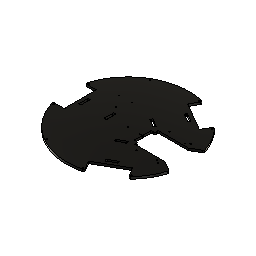
LowerPlate v13 (Autodesk Fusion 360 design; units mm, degrees)
Autodesk Fusion 360 part; units mm, degrees
(part 1 of 2)
sketch "Sketch1" plane through (0, 0, 0) normal (0, 0, 1) x (1, 0, 0)
  line L0 (0, 0) -> (-132.5, 0) construction
  line L1 (0, 0) -> (132.5, 0) construction
  line L2 (0, 0) -> (66.25, 114.7484) construction
  line L3 (0, 0) -> (66.25, -114.7484) construction
  line L4 (-127.7938, -35) -> (-103.7938, -35) construction
  line L5 (-103.7938, -35) -> (-103.7938, 35) construction
  line L6 (-103.7938, 35) -> (-127.7938, 35) construction
  line L7 (-127.7938, 35) -> (-127.7938, -35) construction
  line L8 (-103.7938, 35) -> (-104.8544, 33.9393) construction
  line L9 (-103.7938, -35) -> (-104.8544, -33.9393) construction
  arc A0 (-124.4739, -35) -> (-126.8676, -38.2212) centre (-124.4739, -37.5) ccw
  arc A1 (-126.8676, -38.2212) -> (-124.4739, -35) centre (-124.4739, -37.5) ccw construction
  arc A2 (-103.7938, -35) -> (-103.7938, -32.8787) centre (-104.8544, -33.9393) ccw
  arc A3 (-103.7938, -32.8787) -> (-105.9151, -35) centre (-104.8544, -33.9393) ccw construction
  arc A4 (-105.9151, -35) -> (-103.7938, -35) centre (-104.8544, -33.9393) ccw
  arc A5 (-103.7938, 32.8787) -> (-105.9151, 35) centre (-104.8544, 33.9393) ccw
  arc A6 (-105.9151, 35) -> (-103.7938, 32.8787) centre (-104.8544, 33.9393) ccw construction
  arc A7 (-126.8676, 38.2212) -> (-124.4739, 35) centre (-124.4739, 37.5) ccw
  arc A8 (-124.4739, 35) -> (-126.8676, 38.2212) centre (-124.4739, 37.5) ccw construction
  line L10 (-124.4739, 35) -> (-105.9151, 35)
  line L11 (-103.7938, 32.8787) -> (-103.7938, -32.8787)
  line L12 (-105.9151, -35) -> (-124.4739, -35)
  line L13 (33.586, 128.1727) -> (94.2078, 93.1727) construction
  line L14 (33.586, 128.1727) -> (21.586, 107.388) construction
  line L15 (21.586, 107.388) -> (82.2078, 72.388) construction
  line L16 (82.2078, 72.388) -> (94.2078, 93.1727) construction
  arc A9 (31.9261, 125.2976) -> (30.3332, 128.9812) centre (29.761, 126.5476) ccw
  arc A10 (30.3332, 128.9812) -> (31.9261, 125.2976) centre (29.761, 126.5476) ccw construction
  arc A11 (96.5343, 90.76) -> (92.5478, 90.2976) centre (94.7129, 89.0476) ccw
  arc A12 (92.5478, 90.2976) -> (96.5343, 90.76) centre (94.7129, 89.0476) ccw construction
  line L17 (21.586, 107.388) -> (23.0349, 107.7763) construction
  arc A13 (22.6467, 109.2252) -> (23.4231, 106.3274) centre (23.0349, 107.7763) ccw
  arc A14 (23.4231, 106.3274) -> (22.6467, 109.2252) centre (23.0349, 107.7763) ccw construction
  line L18 (82.2078, 72.388) -> (81.8196, 73.8369) construction
  arc A15 (80.3707, 73.4487) -> (83.2684, 74.2252) centre (81.8196, 73.8369) ccw
  arc A16 (83.2684, 74.2252) -> (80.3707, 73.4487) centre (81.8196, 73.8369) ccw construction
  line L19 (83.2684, 74.2252) -> (92.5478, 90.2976)
  line L20 (80.3707, 73.4487) -> (23.4231, 106.3274)
  line L21 (22.6467, 109.2252) -> (31.9261, 125.2976)
  line L22 (33.586, -128.1727) -> (94.2078, -93.1727) construction
  line L23 (33.586, -128.1727) -> (21.586, -107.388) construction
  line L24 (21.586, -107.388) -> (82.2078, -72.388) construction
  line L25 (82.2078, -72.388) -> (94.2078, -93.1727) construction
  line L26 (82.2078, -72.388) -> (81.8196, -73.8369) construction
  line L27 (21.586, -107.388) -> (23.0349, -107.7763) construction
  arc A17 (23.4231, -106.3274) -> (22.6467, -109.2252) centre (23.0349, -107.7763) ccw
  arc A18 (22.6467, -109.2252) -> (23.4231, -106.3274) centre (23.0349, -107.7763) ccw construction
  arc A19 (83.2684, -74.2252) -> (80.3707, -73.4487) centre (81.8196, -73.8369) ccw
  arc A20 (80.3707, -73.4487) -> (83.2684, -74.2252) centre (81.8196, -73.8369) ccw construction
  arc A21 (92.5478, -90.2976) -> (96.5343, -90.76) centre (94.7129, -89.0476) ccw
  arc A22 (96.5343, -90.76) -> (92.5478, -90.2976) centre (94.7129, -89.0476) ccw construction
  arc A23 (30.3333, -128.9812) -> (31.9261, -125.2976) centre (29.761, -126.5476) ccw
  arc A24 (31.9261, -125.2976) -> (30.3333, -128.9812) centre (29.761, -126.5476) ccw construction
  line L28 (92.5478, -90.2976) -> (83.2684, -74.2252)
  line L29 (80.3707, -73.4487) -> (23.4231, -106.3274)
  line L30 (22.6467, -109.2252) -> (31.9261, -125.2976)
  arc A25 (30.3332, 128.9812) -> (-126.8676, 38.2212) centre (0, 0) ccw
  arc A26 (-126.8676, 38.2212) -> (-126.8676, -38.2212) centre (0, 0) ccw construction
  arc A27 (30.3333, -128.9812) -> (30.3332, 128.9812) centre (0, 0) ccw construction
  arc A28 (-126.8676, -38.2212) -> (30.3333, -128.9812) centre (0, 0) ccw
  line L31 (-103.7938, 18.4) -> (-19.3938, 18.4) construction
  line L32 (-19.3938, 18.4) -> (-19.3938, -18.4) construction
  line L33 (-19.3938, -18.4) -> (-103.7938, -18.4) construction
  line L34 (-96.7938, 10) -> (-91.9938, 10) construction
  line L35 (-91.9938, 10) -> (-91.9938, -10) construction
  line L36 (-91.9938, -10) -> (-96.7938, -10) construction
  line L37 (-96.7938, -10) -> (-96.7938, 10) construction
  line L38 (-96.7938, 10) -> (-91.9938, -10) construction
  line L39 (-41.9938, 10) -> (-37.1938, 10) construction
  line L40 (-37.1938, 10) -> (-37.1938, -10) construction
  line L41 (-37.1938, -10) -> (-41.9938, -10) construction
  line L42 (-41.9938, -10) -> (-41.9938, 10) construction
  line L43 (-41.9938, 10) -> (-37.1938, -10) construction
  line L44 (-96.7938, 10) -> (-95.7331, 8.9393) construction
  line L45 (-91.9938, 10) -> (-93.0544, 8.9393) construction
  line L46 (-96.7938, -10) -> (-95.7331, -8.9393) construction
  line L47 (-91.9938, -10) -> (-93.0544, -8.9393) construction
  arc A29 (-94.1151, 10) -> (-91.9938, 7.8787) centre (-93.0544, 8.9393) ccw construction
  arc A30 (-91.9938, 7.8787) -> (-91.9938, 10) centre (-93.0544, 8.9393) ccw
  arc A31 (-91.9938, 10) -> (-94.1151, 10) centre (-93.0544, 8.9393) ccw
  arc A32 (-96.7938, 7.8787) -> (-94.6725, 10) centre (-95.7331, 8.9393) ccw construction
  arc A33 (-94.6725, 10) -> (-96.7938, 10) centre (-95.7331, 8.9393) ccw
  arc A34 (-96.7938, 10) -> (-96.7938, 7.8787) centre (-95.7331, 8.9393) ccw
  arc A35 (-94.6725, -10) -> (-96.7938, -7.8787) centre (-95.7331, -8.9393) ccw construction
  arc A36 (-96.7938, -7.8787) -> (-96.7938, -10) centre (-95.7331, -8.9393) ccw
  arc A37 (-96.7938, -10) -> (-94.6725, -10) centre (-95.7331, -8.9393) ccw
  arc A38 (-91.9938, -7.8787) -> (-94.1151, -10) centre (-93.0544, -8.9393) ccw construction
  arc A39 (-94.1151, -10) -> (-91.9938, -10) centre (-93.0544, -8.9393) ccw
  arc A40 (-91.9938, -10) -> (-91.9938, -7.8787) centre (-93.0544, -8.9393) ccw
  line L48 (-94.6725, 10) -> (-94.1151, 10)
  line L49 (-96.7938, 7.8787) -> (-96.7938, -7.8787)
  line L50 (-91.9938, -7.8787) -> (-91.9938, 7.8787)
  line L51 (-94.6725, -10) -> (-94.1151, -10)
  line L52 (-41.9938, 10) -> (-40.9331, 8.9393) construction
  line L53 (-37.1938, 10) -> (-38.2544, 8.9393) construction
  line L54 (-41.9938, -10) -> (-40.9331, -8.9393) construction
  line L55 (-37.1938, -10) -> (-38.2544, -8.9393) construction
  arc A41 (-37.1938, -7.8787) -> (-39.3151, -10) centre (-38.2544, -8.9393) ccw construction
  arc A42 (-39.3151, -10) -> (-37.1938, -10) centre (-38.2544, -8.9393) ccw
  arc A43 (-37.1938, -10) -> (-37.1938, -7.8787) centre (-38.2544, -8.9393) ccw
  arc A44 (-39.8725, -10) -> (-41.9938, -7.8787) centre (-40.9331, -8.9393) ccw construction
  arc A45 (-41.9938, -10) -> (-39.8725, -10) centre (-40.9331, -8.9393) ccw
  arc A46 (-41.9938, -7.8787) -> (-41.9938, -10) centre (-40.9331, -8.9393) ccw
  arc A47 (-41.9938, 7.8787) -> (-39.8725, 10) centre (-40.9331, 8.9393) ccw construction
  arc A48 (-41.9938, 10) -> (-41.9938, 7.8787) centre (-40.9331, 8.9393) ccw
  arc A49 (-39.8725, 10) -> (-41.9938, 10) centre (-40.9331, 8.9393) ccw
  arc A50 (-39.3151, 10) -> (-37.1938, 7.8787) centre (-38.2544, 8.9393) ccw construction
  arc A51 (-37.1938, 10) -> (-39.3151, 10) centre (-38.2544, 8.9393) ccw
  arc A52 (-37.1938, 7.8787) -> (-37.1938, 10) centre (-38.2544, 8.9393) ccw
  line L56 (-39.8725, -10) -> (-39.3151, -10)
  line L57 (-37.1938, -7.8787) -> (-37.1938, 7.8787)
  line L58 (-41.9938, 7.8787) -> (-41.9938, -7.8787)
  line L59 (-39.8725, 10) -> (-39.3151, 10)
  line L60 (35.962, 99.088) -> (-6.238, 25.9955) construction
  line L61 (-6.238, 25.9955) -> (25.6318, 7.5955) construction
  line L62 (25.6318, 7.5955) -> (67.8318, 80.688) construction
  line L63 (39.7366, 88.8259) -> (57.0571, 78.8259) construction
  line L64 (57.0571, 78.8259) -> (54.6571, 74.6689) construction
  line L65 (54.6571, 74.6689) -> (37.3366, 84.6689) construction
  line L66 (37.3366, 84.6689) -> (39.7366, 88.8259) construction
  line L67 (39.7366, 88.8259) -> (54.6571, 74.6689) construction
  line L68 (12.3366, 41.3677) -> (29.6571, 31.3677) construction
  line L69 (29.6571, 31.3677) -> (27.2571, 27.2108) construction
  line L70 (27.2571, 27.2108) -> (9.9366, 37.2108) construction
  line L71 (9.9366, 37.2108) -> (12.3366, 41.3677) construction
  line L72 (12.3366, 41.3677) -> (27.2571, 27.2108) construction
  line L73 (37.3366, 84.6689) -> (38.7855, 85.0572) construction
  line L74 (39.7366, 88.8259) -> (40.1249, 87.377) construction
  line L75 (54.6571, 74.6689) -> (54.2689, 76.1178) construction
  line L76 (57.0571, 78.8259) -> (55.6083, 78.4376) construction
  arc A53 (55.22, 79.8865) -> (55.9965, 76.9888) centre (55.6083, 78.4376) ccw construction
  arc A54 (55.9965, 76.9888) -> (57.0571, 78.8259) centre (55.6083, 78.4376) ccw
  arc A55 (57.0571, 78.8259) -> (55.22, 79.8865) centre (55.6083, 78.4376) ccw
  arc A56 (55.7178, 76.5061) -> (52.82, 75.7296) centre (54.2689, 76.1178) ccw construction
  arc A57 (54.6571, 74.6689) -> (55.7178, 76.5061) centre (54.2689, 76.1178) ccw
  arc A58 (52.82, 75.7296) -> (54.6571, 74.6689) centre (54.2689, 76.1178) ccw
  arc A59 (39.1738, 83.6083) -> (38.3973, 86.5061) centre (38.7855, 85.0572) ccw construction
  arc A60 (37.3366, 84.6689) -> (39.1738, 83.6083) centre (38.7855, 85.0572) ccw
  arc A61 (38.3973, 86.5061) -> (37.3366, 84.6689) centre (38.7855, 85.0572) ccw
  arc A62 (38.676, 86.9888) -> (41.5738, 87.7652) centre (40.1249, 87.377) ccw construction
  arc A63 (41.5738, 87.7652) -> (39.7366, 88.8259) centre (40.1249, 87.377) ccw
  arc A64 (39.7366, 88.8259) -> (38.676, 86.9888) centre (40.1249, 87.377) ccw
  line L77 (38.3973, 86.5061) -> (38.676, 86.9888)
  line L78 (41.5738, 87.7652) -> (55.22, 79.8865)
  line L79 (55.9965, 76.9888) -> (55.7178, 76.5061)
  line L80 (52.82, 75.7296) -> (39.1738, 83.6083)
  line L81 (9.9366, 37.2108) -> (11.3855, 37.599) construction
  line L82 (12.3366, 41.3677) -> (12.7249, 39.9188) construction
  line L83 (27.2571, 27.2108) -> (26.8689, 28.6596) construction
  line L84 (29.6571, 31.3677) -> (28.2083, 30.9795) construction
  arc A65 (11.276, 39.5306) -> (14.1738, 40.307) centre (12.7249, 39.9188) ccw construction
  arc A66 (14.1738, 40.307) -> (12.3366, 41.3677) centre (12.7249, 39.9188) ccw
  arc A67 (12.3366, 41.3677) -> (11.276, 39.5306) centre (12.7249, 39.9188) ccw
  arc A68 (11.7738, 36.1501) -> (10.9973, 39.0479) centre (11.3855, 37.599) ccw construction
  arc A69 (10.9973, 39.0479) -> (9.9366, 37.2108) centre (11.3855, 37.599) ccw
  arc A70 (9.9366, 37.2108) -> (11.7738, 36.1501) centre (11.3855, 37.599) ccw
  arc A71 (28.3178, 29.0479) -> (25.42, 28.2714) centre (26.8689, 28.6596) ccw construction
  arc A72 (25.42, 28.2714) -> (27.2571, 27.2108) centre (26.8689, 28.6596) ccw
  arc A73 (27.2571, 27.2108) -> (28.3178, 29.0479) centre (26.8689, 28.6596) ccw
  arc A74 (27.82, 32.4283) -> (28.5965, 29.5306) centre (28.2083, 30.9795) ccw construction
  arc A75 (28.5965, 29.5306) -> (29.6571, 31.3677) centre (28.2083, 30.9795) ccw
  arc A76 (29.6571, 31.3677) -> (27.82, 32.4283) centre (28.2083, 30.9795) ccw
  line L85 (10.9973, 39.0479) -> (11.276, 39.5306)
  line L86 (11.7738, 36.1501) -> (25.42, 28.2714)
  line L87 (28.3178, 29.0479) -> (28.5965, 29.5306)
  line L88 (27.82, 32.4283) -> (14.1738, 40.307)
  line L89 (35.962, -99.088) -> (-6.238, -25.9955) construction
  line L90 (-6.238, -25.9955) -> (25.6318, -7.5955) construction
  line L91 (25.6318, -7.5955) -> (67.8318, -80.688) construction
  line L92 (39.7366, -88.8259) -> (57.0571, -78.8259) construction
  line L93 (57.0571, -78.8259) -> (54.6571, -74.6689) construction
  line L94 (54.6571, -74.6689) -> (37.3366, -84.6689) construction
  line L95 (37.3366, -84.6689) -> (39.7366, -88.8259) construction
  line L96 (37.3366, -84.6689) -> (57.0571, -78.8259) construction
  line L97 (12.3366, -41.3677) -> (29.6571, -31.3677) construction
  line L98 (29.6571, -31.3677) -> (27.2571, -27.2108) construction
  line L99 (27.2571, -27.2108) -> (9.9366, -37.2108) construction
  line L100 (9.9366, -37.2108) -> (12.3366, -41.3677) construction
  line L101 (9.9366, -37.2108) -> (29.6571, -31.3677) construction
  line L102 (9.9366, -37.2108) -> (11.3855, -37.599) construction
  line L103 (12.3366, -41.3677) -> (12.7249, -39.9188) construction
  line L104 (27.2571, -27.2108) -> (26.8689, -28.6596) construction
  line L105 (29.6571, -31.3677) -> (28.2083, -30.9795) construction
  arc A77 (25.42, -28.2714) -> (28.3178, -29.0479) centre (26.8689, -28.6596) ccw construction
  arc A78 (28.3178, -29.0479) -> (27.2571, -27.2108) centre (26.8689, -28.6596) ccw
  arc A79 (27.2571, -27.2108) -> (25.42, -28.2714) centre (26.8689, -28.6596) ccw
  arc A80 (28.5965, -29.5306) -> (27.82, -32.4283) centre (28.2083, -30.9795) ccw construction
  arc A81 (29.6571, -31.3677) -> (28.5965, -29.5306) centre (28.2083, -30.9795) ccw
  arc A82 (27.82, -32.4283) -> (29.6571, -31.3677) centre (28.2083, -30.9795) ccw
  arc A83 (14.1738, -40.307) -> (11.276, -39.5306) centre (12.7249, -39.9188) ccw construction
  arc A84 (12.3366, -41.3677) -> (14.1738, -40.307) centre (12.7249, -39.9188) ccw
  arc A85 (11.276, -39.5306) -> (12.3366, -41.3677) centre (12.7249, -39.9188) ccw
  arc A86 (10.9973, -39.0479) -> (11.7738, -36.1501) centre (11.3855, -37.599) ccw construction
  arc A87 (9.9366, -37.2108) -> (10.9973, -39.0479) centre (11.3855, -37.599) ccw
  arc A88 (11.7738, -36.1501) -> (9.9366, -37.2108) centre (11.3855, -37.599) ccw
  line L106 (28.5965, -29.5306) -> (28.3178, -29.0479)
  line L107 (25.42, -28.2714) -> (11.7738, -36.1501)
  line L108 (27.82, -32.4283) -> (14.1738, -40.307)
  line L109 (11.276, -39.5306) -> (10.9973, -39.0479)
  line L110 (37.3366, -84.6689) -> (38.7855, -85.0572) construction
  line L111 (39.7366, -88.8259) -> (40.1249, -87.377) construction
  line L112 (54.6571, -74.6689) -> (54.2689, -76.1178) construction
  line L113 (57.0571, -78.8259) -> (55.6083, -78.4376) construction
  arc A89 (38.3973, -86.5061) -> (39.1738, -83.6083) centre (38.7855, -85.0572) ccw construction
  arc A90 (39.1738, -83.6083) -> (37.3366, -84.6689) centre (38.7855, -85.0572) ccw
  arc A91 (37.3366, -84.6689) -> (38.3973, -86.5061) centre (38.7855, -85.0572) ccw
  arc A92 (41.5738, -87.7652) -> (38.676, -86.9888) centre (40.1249, -87.377) ccw construction
  arc A93 (38.676, -86.9888) -> (39.7366, -88.8259) centre (40.1249, -87.377) ccw
  arc A94 (39.7366, -88.8259) -> (41.5738, -87.7652) centre (40.1249, -87.377) ccw
  arc A95 (55.9965, -76.9888) -> (55.22, -79.8865) centre (55.6083, -78.4376) ccw construction
  arc A96 (55.22, -79.8865) -> (57.0571, -78.8259) centre (55.6083, -78.4376) ccw
  arc A97 (57.0571, -78.8259) -> (55.9965, -76.9888) centre (55.6083, -78.4376) ccw
  arc A98 (52.82, -75.7296) -> (55.7178, -76.5061) centre (54.2689, -76.1178) ccw construction
  arc A99 (55.7178, -76.5061) -> (54.6571, -74.6689) centre (54.2689, -76.1178) ccw
  arc A100 (54.6571, -74.6689) -> (52.82, -75.7296) centre (54.2689, -76.1178) ccw
  line L114 (38.676, -86.9888) -> (38.3973, -86.5061)
  line L115 (39.1738, -83.6083) -> (52.82, -75.7296)
  line L116 (55.7178, -76.5061) -> (55.9965, -76.9888)
  line L117 (55.22, -79.8865) -> (41.5738, -87.7652)
  line L118 (32, 18.3) -> (131.2302, 18.3) construction
  line L119 (131.2302, 18.3) -> (131.2302, -18.3) construction
  line L120 (131.2302, -18.3) -> (32, -18.3) construction
  line L121 (32, -18.3) -> (32, 18.3) construction
  line L122 (40, 25.5) -> (130.0231, 25.5) construction
  line L123 (130.0231, 25.5) -> (130.0231, -25.5) construction
  line L124 (130.0231, -25.5) -> (40, -25.5) construction
  line L125 (40, -25.5) -> (40, 25.5) construction
  line L126 (100, 25.5) -> (100, -25.5) construction
  line L127 (100, 22.5) -> (126.9212, 38.0429) construction
  line L128 (100, -22.5) -> (126.9212, -38.0429) construction
  line L129 (32, -18.3) -> (33.0607, -17.2393) construction
  line L130 (40, -25.5) -> (41.0607, -24.4393) construction
  circle A101 centre (33.0607, -17.2393) radius 1.5 construction
  circle A102 centre (41.0607, -24.4393) radius 1.5 construction
  circle A103 centre (37.5, -20.8) radius 2.5 construction
  line L131 (32, 18.3) -> (33.0607, 17.2393) construction
  line L132 (40, 25.5) -> (41.0607, 24.4393) construction
  circle A104 centre (41.0607, 24.4393) radius 1.5 construction
  circle A105 centre (33.0607, 17.2393) radius 1.5 construction
  circle A106 centre (37.5, 20.8) radius 2.5 construction
  circle A107 centre (123.9454, -39.2116) radius 2.5 construction
  circle A108 centre (123.9454, 39.2116) radius 2.5 construction
  circle A109 centre (104.5263, 28) radius 2.5 construction
  circle A110 centre (104.5263, -28) radius 2.5 construction
  line L133 (32, 16.1787) -> (32, -16.1787)
  line L134 (34.1213, -18.3) -> (37.5, -18.3)
  line L135 (40, -20.8) -> (40, -23.3787)
  line L136 (42.1213, -25.5) -> (104.5263, -25.5)
  line L137 (105.7763, -25.8349) -> (125.1954, -37.0465)
  line L138 (34.1213, 18.3) -> (37.5, 18.3)
  line L139 (40, 20.8) -> (40, 23.3787)
  line L140 (42.1213, 25.5) -> (104.5263, 25.5)
  line L141 (105.7763, 25.8349) -> (125.1954, 37.0465)
  arc A111 (34.1213, 18.3) -> (32, 16.1787) centre (33.0607, 17.2393) ccw
  arc A112 (42.1213, 25.5) -> (40, 23.3787) centre (41.0607, 24.4393) ccw
  arc A113 (32, -16.1787) -> (34.1213, -18.3) centre (33.0607, -17.2393) ccw
  arc A114 (40, -23.3787) -> (42.1213, -25.5) centre (41.0607, -24.4393) ccw
  arc A115 (37.5, 18.3) -> (40, 20.8) centre (37.5, 20.8) ccw
  arc A116 (40, -20.8) -> (37.5, -18.3) centre (37.5, -20.8) ccw
  arc A117 (104.5263, 25.5) -> (105.7763, 25.8349) centre (104.5263, 28) ccw
  arc A118 (105.7763, -25.8349) -> (104.5263, -25.5) centre (104.5263, -28) ccw
  line L142 (0, 0) -> (123.9454, -39.2116) construction
  line L143 (123.9454, -39.2116) -> (126.3289, -39.9657) construction
  arc A119 (126.3289, -39.9657) -> (125.1954, -37.0465) centre (123.9454, -39.2116) ccw
  line L144 (0, 0) -> (123.9454, 39.2116) construction
  line L145 (123.9454, 39.2116) -> (126.3289, 39.9657) construction
  arc A120 (125.1954, 37.0465) -> (126.3289, 39.9657) centre (123.9454, 39.2116) ccw
  arc A121 (96.5343, -90.76) -> (126.3289, -39.9657) centre (0, 0) ccw
  arc A122 (126.3289, 39.9657) -> (96.5343, 90.76) centre (0, 0) ccw
  line L146 (126.9212, -38.0429) -> (122.7474, -39.6747) construction
  circle A123 centre (122.7474, -39.6747) radius 3.5 construction
  circle A124 centre (122.7474, -39.6747) radius 1.5 construction
  line L147 (94.2078, -93.1727) -> (94.9024, -87.3758) construction
  circle A125 centre (94.9024, -87.3758) radius 3.5 construction
  circle A126 centre (94.9024, -87.3758) radius 1.5
  line L148 (33.586, -128.1727) -> (28.2185, -125.8758) construction
  circle A127 centre (28.2185, -125.8758) radius 3.5 construction
  circle A128 centre (28.2185, -125.8758) radius 1.5
  line L149 (-127.7938, -35) -> (-123.1209, -38.5) construction
  circle A129 centre (-123.1209, -38.5) radius 3.5 construction
  circle A130 centre (-123.1209, -38.5) radius 1.5
  line L150 (-127.7938, 35) -> (-123.1209, 38.5) construction
  circle A131 centre (-123.1209, 38.5) radius 3.5 construction
  circle A132 centre (-123.1209, 38.5) radius 1.5
  line L151 (33.586, 128.1727) -> (28.2185, 125.8758) construction
  circle A133 centre (28.2185, 125.8758) radius 3.5 construction
  circle A134 centre (28.2185, 125.8758) radius 1.5
  line L152 (94.2078, 93.1727) -> (94.9024, 87.3758) construction
  circle A135 centre (94.9024, 87.3758) radius 3.5 construction
  circle A136 centre (94.9024, 87.3758) radius 1.5
  line L153 (126.9212, 38.0429) -> (122.7474, 39.6747) construction
  circle A137 centre (122.7474, 39.6747) radius 3.5 construction
  circle A138 centre (122.7474, 39.6747) radius 1.5 construction
  line L154 (-123.1209, -38.5) -> (28.2185, -125.8758) construction
  line L155 (-123.1209, 38.5) -> (28.2185, 125.8758) construction
  line L156 (0, 0) -> (-47.4512, -82.1879) construction
  line L157 (-47.4512, -82.1879) -> (-64.5, -111.7173) construction
  circle A139 centre (-64.5, -111.7173) radius 3.5 construction
  circle A140 centre (-64.5, -111.7173) radius 1.5
  line L158 (0, 0) -> (-47.4512, 82.1879) construction
  line L159 (-47.4512, 82.1879) -> (-64.5, 111.7173) construction
  circle A141 centre (-64.5, 111.7173) radius 3.5 construction
  circle A142 centre (-64.5, 111.7173) radius 1.5
  circle A143 centre (100, -35.5) radius 1.5
  line L160 (100, -25.5) -> (100, -35.5) construction
  line L161 (100, 25.5) -> (100, 35.5) construction
  circle A144 centre (100, 35.5) radius 1.5
  circle A145 centre (53.2894, -35.5) radius 1.5
  circle A146 centre (53.2894, 35.5) radius 1.5
  point P0 (-19.3938, 0)
  point P1 (-94.3938, 0)
  point P2 (-39.5938, 0)
  point P3 (9.6969, 16.7955)
  point P4 (47.1969, 81.7474)
  point P5 (19.7969, 34.2892)
  point P6 (9.6969, -16.7955)
  point P7 (47.1969, -81.7474)
  point P8 (19.7969, -34.2892)
  point P9 (-47.4512, 82.1879)
  point P10 (-47.4512, -82.1879)
  dimension "d1" = 265
  dimension "d2" = 60
  dimension "d3" = 60
  dimension "d4" = 24
  dimension "d5" = 70
  dimension "d6" = 5
  dimension "d7" = 1.5
  dimension "d8" = 45
  dimension "d9" = 1.5
  dimension "d10" = 45
  dimension "d11" = 5
  dimension "d12" = 70
  dimension "d13" = 24
  dimension "d14" = 5
  dimension "d15" = 5
  dimension "d16" = 1.5
  dimension "d17" = 45
  dimension "d18" = 1.5
  dimension "d19" = 45
  dimension "d21" = 70
  dimension "d22" = 24
  dimension "d23" = 5
  dimension "d24" = 5
  dimension "d25" = 1.5
  dimension "d26" = 45
  dimension "d27" = 1.5
  dimension "d28" = 45
  dimension "d29" = 36.8
  dimension "d30" = 108.4
  dimension "d31" = 4.8
  dimension "d32" = 20
  dimension "d34" = 72.6
  dimension "d35" = 4.8
  dimension "d36" = 20
  dimension "d37" = 50
  dimension "d38" = 1.5
  dimension "d39" = 1.5
  dimension "d40" = 1.5
  dimension "d41" = 1.5
  dimension "d42" = 45
  dimension "d43" = 45
  dimension "d44" = 45
  dimension "d45" = 45
  dimension "d46" = 1.5
  dimension "d47" = 1.5
  dimension "d48" = 1.5
  dimension "d49" = 1.5
  dimension "d50" = 45
  dimension "d51" = 45
  dimension "d52" = 45
  dimension "d53" = 45
  dimension "d54" = 36.8
  dimension "d55" = 108.4
  dimension "d56" = 4.8
  dimension "d57" = 20
  dimension "d58" = 72.6
  dimension "d59" = 4.8
  dimension "d60" = 20
  dimension "d61" = 50
  dimension "d62" = 1.5
  dimension "d63" = 1.5
  dimension "d64" = 1.5
  dimension "d65" = 1.5
  dimension "d66" = 45
  dimension "d67" = 45
  dimension "d68" = 45
  dimension "d69" = 45
  dimension "d70" = 1.5
  dimension "d71" = 1.5
  dimension "d72" = 1.5
  dimension "d73" = 1.5
  dimension "d74" = 45
  dimension "d75" = 45
  dimension "d76" = 45
  dimension "d77" = 45
  dimension "d78" = 36.8
  dimension "d79" = 108.4
  dimension "d81" = 4.8
  dimension "d82" = 20
  dimension "d83" = 72.6
  dimension "d84" = 4.8
  dimension "d85" = 20
  dimension "d86" = 50
  dimension "d87" = 1.5
  dimension "d88" = 1.5
  dimension "d89" = 1.5
  dimension "d90" = 1.5
  dimension "d91" = 45
  dimension "d92" = 45
  dimension "d93" = 45
  dimension "d94" = 45
  dimension "d95" = 1.5
  dimension "d96" = 1.5
  dimension "d97" = 1.5
  dimension "d98" = 1.5
  dimension "d99" = 45
  dimension "d100" = 45
  dimension "d101" = 45
  dimension "d102" = 45
  dimension "d103" = 36.6
  dimension "d104" = 32
  dimension "d105" = 8
  dimension "d106" = 51
  dimension "d107" = 60
  dimension "d108" = 3
  dimension "d109" = 30
  dimension "d110" = 3
  dimension "d111" = 30
  dimension "d112" = 1.5
  dimension "d113" = 1.5
  dimension "d114" = 45
  dimension "d115" = 45
  dimension "d116" = 5
  dimension "d117" = 1.5
  dimension "d118" = 1.5
  dimension "d119" = 45
  dimension "d120" = 45
  dimension "d121" = 5
  dimension "d122" = 5
  dimension "d123" = 5
  dimension "d124" = 5
  dimension "d125" = 5
  dimension "d131" = 7
  dimension "d132" = 3
  dimension "d133" = 7
  dimension "d134" = 3
  dimension "d135" = 7
  dimension "d136" = 3
  dimension "d137" = 7
  dimension "d138" = 3
  dimension "d139" = 7
  dimension "d140" = 3
  dimension "d141" = 7
  dimension "d142" = 3
  dimension "d143" = 7
  dimension "d144" = 3
  dimension "d145" = 7
  dimension "d146" = 3
  dimension "d147" = 7
  dimension "d148" = 3
  dimension "d149" = 7
  dimension "d150" = 3
  dimension "d189" = 3
  dimension "d190" = 10
  dimension "d191" = 10
  dimension "d192" = 3
  dimension "d193" = 3
  dimension "d194" = 10
  dimension "d195" = 10
  dimension "d196" = 3
  dimension "d197" = 10
  dimension "d198" = 10
  constraint coincident L0.start L1.start
  constraint coincident L0.end A26
  constraint horizontal L0
  constraint coincident L1.end A26
  constraint parallel L0 L1
  constraint coincident L2.end A26
  constraint coincident L3.end A26
  constraint horizontal L4
  constraint vertical L5
  constraint horizontal L6
  constraint vertical L7
  constraint coincident L4.start A26
  constraint coincident L6.end A26
  constraint tangent L6 A7
  constraint tangent A7 A26
  constraint coincident L8.end A5.centre
  constraint coincident L5.end A5
  constraint coincident L9.end A2.centre
  constraint tangent L4 A0
  constraint tangent A0 A26
  constraint coincident L4 A0.start
  constraint concentric A0 A1
  constraint coincident L5 A2.end
  constraint coincident L4 A3.end
  constraint concentric A2 A3
  constraint concentric A2 A4
  constraint coincident L6 A5.end
  constraint coincident L5 A5.start
  constraint concentric A5 A6
  constraint coincident L6 A7.end
  constraint concentric A7 A8
  constraint coincident L13.start A26
  constraint coincident L13.end A26
  constraint perpendicular L2 L13
  constraint perpendicular L13 L14
  constraint perpendicular L14 L15
  constraint perpendicular L15 L16
  constraint tangent L14 A9
  constraint tangent A9 A26
  constraint coincident L14 A9.start
  constraint concentric A9 A10
  constraint tangent A11 A26
  constraint tangent L16 A11
  constraint coincident L16 A11.end
  constraint coincident A11.start A26
  constraint concentric A11 A12
  constraint coincident L17.end A13.centre
  constraint coincident L14.end A13
  constraint coincident L15 A13.end
  constraint coincident L14 A13.start
  constraint concentric A13 A14
  constraint coincident L18.end A15.centre
  constraint coincident L15.end A15
  constraint coincident L16 A15.end
  constraint coincident L15 A15.start
  constraint concentric A15 A16
  constraint coincident L22.start A26
  constraint coincident L22.end A26
  constraint perpendicular L3 L22
  constraint perpendicular L22 L23
  constraint perpendicular L23 L24
  constraint perpendicular L24 L25
  constraint tangent L23 A23
  constraint tangent A23 A26
  constraint tangent L25 A21
  constraint tangent A21 A26
  constraint coincident L26.end A19.centre
  constraint coincident L24.end A19
  constraint coincident L27.end A17.centre
  constraint coincident L23.end A17
  constraint coincident L23 A17.end
  constraint coincident L24 A17.start
  constraint concentric A17 A18
  constraint coincident L24 A19.end
  constraint coincident L25 A19.start
  constraint concentric A19 A20
  constraint coincident A21.end A26
  constraint coincident L25 A21.start
  constraint concentric A21 A22
  constraint coincident L23 A23.end
  constraint coincident A23.start A26
  constraint concentric A23 A24
  constraint coincident A21 A22.end
  constraint concentric A25 A26
  constraint concentric A26 A27
  constraint concentric A26 A28
  constraint coincident L11 L31.start
  constraint perpendicular L11 L31
  constraint perpendicular L31 L32
  constraint coincident L11 L33.end
  constraint perpendicular L32 L33
  constraint midpoint L32 P0
  constraint coincident L0 P0
  constraint horizontal L34
  constraint vertical L35
  constraint horizontal L36
  constraint vertical L37
  constraint midpoint L38 P1
  constraint coincident L0 P1
  constraint horizontal L39
  constraint vertical L40
  constraint horizontal L41
  constraint vertical L42
  constraint midpoint L43 P2
  constraint coincident L0 P2
  constraint coincident L44.end A32.centre
  constraint coincident L45.end A29.centre
  constraint coincident L46.end A35.centre
  constraint coincident L47.end A38.centre
  constraint coincident L35 A29.end
  constraint concentric A29 A30
  constraint coincident L34 A29.start
  constraint concentric A29 A31
  constraint coincident L34 A32.end
  constraint concentric A32 A33
  constraint coincident L37 A32.start
  constraint concentric A32 A34
  constraint coincident L37 A35.end
  constraint concentric A35 A36
  constraint coincident L36 A35.start
  constraint concentric A35 A37
  constraint coincident L36 A38.end
  constraint concentric A38 A39
  constraint coincident L35 A38.start
  constraint concentric A38 A40
  constraint coincident L54.end A44.centre
  constraint coincident L55.end A41.centre
  constraint coincident L52.end A47.centre
  constraint coincident L53.end A50.centre
  constraint coincident L41 A41.end
  constraint concentric A41 A42
  constraint coincident L40 A41.start
  constraint concentric A41 A43
  constraint coincident L41 A44.start
  constraint concentric A44 A45
  constraint coincident L42 A44.end
  constraint concentric A44 A46
  constraint coincident L42 A47.start
  constraint concentric A47 A48
  constraint coincident L39 A47.end
  constraint concentric A47 A49
  constraint coincident L39 A50.start
  constraint concentric A50 A51
  constraint coincident L40 A50.end
  constraint concentric A50 A52
  constraint coincident L20 L60.start
  constraint perpendicular L20 L60
  constraint perpendicular L60 L61
  constraint coincident L20 L62.end
  constraint perpendicular L61 L62
  constraint midpoint L61 P3
  constraint coincident L2 P3
  constraint perpendicular L2 L63
  constraint perpendicular L63 L64
  constraint perpendicular L64 L65
  constraint perpendicular L65 L66
  constraint midpoint L67 P4
  constraint coincident L2 P4
  constraint perpendicular L2 L68
  constraint perpendicular L68 L69
  constraint perpendicular L2 L70
  constraint perpendicular L70 L71
  constraint midpoint L72 P5
  constraint coincident L2 P5
  constraint coincident L74.end A62.centre
  constraint coincident L73.end A59.centre
  constraint coincident L76.end A53.centre
  constraint coincident L75.end A56.centre
  constraint coincident L64 A53.end
  constraint concentric A53 A54
  constraint coincident L63 A53.start
  constraint concentric A53 A55
  constraint coincident L64 A56.start
  constraint concentric A56 A57
  constraint coincident L65 A56.end
  constraint concentric A56 A58
  constraint coincident L65 A59.start
  constraint concentric A59 A60
  constraint coincident L66 A59.end
  constraint concentric A59 A61
  constraint coincident L63 A62.end
  constraint concentric A62 A63
  constraint coincident L66 A62.start
  constraint concentric A62 A64
  constraint coincident L81.end A68.centre
  constraint coincident L82.end A65.centre
  constraint coincident L84.end A74.centre
  constraint coincident L83.end A71.centre
  constraint coincident L68 A65.end
  constraint concentric A65 A66
  constraint coincident L71 A65.start
  constraint concentric A65 A67
  constraint coincident L71 A68.end
  constraint concentric A68 A69
  constraint coincident L70 A68.start
  constraint concentric A68 A70
  constraint coincident L70 A71.end
  constraint concentric A71 A72
  constraint coincident L69 A71.start
  constraint concentric A71 A73
  constraint coincident L69 A74.end
  constraint concentric A74 A75
  constraint coincident L68 A74.start
  constraint concentric A74 A76
  constraint coincident L29 L89.start
  constraint perpendicular L24 L89
  constraint perpendicular L89 L90
  constraint coincident L24 L91.end
  constraint perpendicular L90 L91
  constraint midpoint L90 P6
  constraint coincident L3 P6
  constraint perpendicular L3 L92
  constraint perpendicular L92 L93
  constraint perpendicular L3 L94
  constraint perpendicular L94 L95
  constraint midpoint L96 P7
  constraint coincident L3 P7
  constraint perpendicular L3 L97
  constraint perpendicular L97 L98
  constraint perpendicular L3 L99
  constraint perpendicular L99 L100
  constraint midpoint L101 P8
  constraint coincident L3 P8
  constraint coincident L102.end A86.centre
  constraint coincident L103.end A83.centre
  constraint coincident L105.end A80.centre
  constraint coincident L104.end A77.centre
  constraint coincident L98 A77.end
  constraint concentric A77 A78
  constraint coincident L99 A77.start
  constraint concentric A77 A79
  constraint coincident L98 A80.start
  constraint concentric A80 A81
  constraint coincident L97 A80.end
  constraint concentric A80 A82
  constraint coincident L97 A83.start
  constraint concentric A83 A84
  constraint coincident L100 A83.end
  constraint concentric A83 A85
  constraint coincident L100 A86.start
  constraint concentric A86 A87
  constraint coincident L99 A86.end
  constraint concentric A86 A88
  constraint coincident L113.end A95.centre
  constraint coincident L112.end A98.centre
  constraint coincident L110.end A89.centre
  constraint coincident L111.end A92.centre
  constraint coincident L94 A89.end
  constraint concentric A89 A90
  constraint coincident L95 A89.start
  constraint concentric A89 A91
  constraint coincident L95 A92.end
  constraint concentric A92 A93
  constraint coincident L92 A92.start
  constraint concentric A92 A94
  constraint coincident L92 A95.end
  constraint concentric A95 A96
  constraint coincident L93 A95.start
  constraint concentric A95 A97
  constraint coincident L93 A98.end
  constraint concentric A98 A99
  constraint coincident L94 A98.start
  constraint concentric A98 A100
  constraint horizontal L118
  constraint vertical L119
  constraint horizontal L120
  constraint vertical L121
  constraint coincident A27 L119.end
  constraint coincident A27 L118.end
  constraint horizontal L122
  constraint vertical L123
  constraint horizontal L124
  constraint vertical L125
  constraint coincident A27 L123.end
  constraint coincident A27 L122.end
  constraint coincident L122 L126.start
  constraint coincident L124 L126.end
  constraint perpendicular L124 L126
  constraint coincident L126 L127.start
  constraint coincident A27 L127.end
  constraint coincident L126 L128.start
  constraint coincident A27 L128.end
  constraint coincident L129.end A101.centre
  constraint coincident L120.end A101
  constraint coincident L130.end A102.centre
  constraint coincident L124.end A102
  constraint tangent L120 A103
  constraint tangent L125 A103
  constraint coincident L132.end A104.centre
  constraint coincident L122.start A104
  constraint coincident L131.end A105.centre
  constraint coincident L118.start A105
  constraint tangent L118 A106
  constraint tangent L125 A106
  constraint tangent L128 A107
  constraint tangent A27 A107
  constraint tangent L127 A108
  constraint tangent A27 A108
  constraint tangent L122 A109
  constraint tangent L127 A109
  constraint tangent L124 A110
  constraint tangent L128 A110
  constraint coincident L121 L133.start
  constraint coincident A105 L133.start
  constraint coincident L121 L133.end
  constraint coincident A101 L133.end
  constraint coincident L120 L134.start
  constraint coincident A101 L134.start
  constraint coincident A103 L134.end
  constraint tangent A103 L134
  constraint coincident A103 L135.start
  constraint coincident A102 L135.end
  constraint coincident L125 L135.end
  constraint tangent A103 L135
  constraint coincident L124 L136.start
  constraint coincident A102 L136.start
  constraint coincident A110 L136.end
  constraint tangent A110 L136
  constraint coincident L128 L137.start
  constraint coincident A110 L137.start
  constraint coincident A107 L137.end
  constraint tangent A107 L137
  constraint coincident L118 L138.start
  constraint coincident A105 L138.start
  constraint coincident L118 L138.end
  constraint coincident A106 L138.end
  constraint coincident L125 L139.start
  constraint coincident A106 L139.start
  constraint coincident L125 L139.end
  constraint coincident A104 L139.end
  constraint coincident L122 L140.start
  constraint coincident A104 L140.start
  constraint coincident L122 L140.end
  constraint coincident A109 L140.end
  constraint coincident L127 L141.start
  constraint coincident A109 L141.start
  constraint coincident A108 L141.end
  constraint tangent A108 L141
  constraint coincident A106.centre A115.centre
  constraint coincident A103.centre A116.centre
  constraint coincident A109.centre A117.centre
  constraint coincident A110.centre A118.centre
  constraint coincident A107.centre L142.end
  constraint coincident A27 L143.end
  constraint coincident A107 L143.end
  constraint parallel L142 L143
  constraint coincident A108.centre L144.end
  constraint coincident A108 L145.end
  constraint parallel L144 L145
  constraint coincident L146.end A123.centre
  constraint tangent A121 A123
  constraint tangent L137 A123
  constraint concentric A123 A124
  constraint coincident L147.end A125.centre
  constraint tangent A27 A125
  constraint tangent L28 A125
  constraint concentric A125 A126
  constraint coincident L148.end A127.centre
  constraint tangent L30 A127
  constraint tangent A28 A127
  constraint concentric A127 A128
  constraint coincident L149.end A129.centre
  constraint tangent A28 A129
  constraint tangent L12 A129
  constraint concentric A129 A130
  constraint coincident L150.end A131.centre
  constraint tangent L10 A131
  constraint tangent A25 A131
  constraint concentric A131 A132
  constraint coincident L151.end A133.centre
  constraint tangent A25 A133
  constraint tangent L21 A133
  constraint concentric A133 A134
  constraint coincident L152.end A135.centre
  constraint tangent A122 A135
  constraint tangent L19 A135
  constraint concentric A135 A136
  constraint coincident L153.end A137.centre
  constraint tangent A122 A137
  constraint tangent L141 A137
  constraint concentric A137 A138
  constraint midpoint L155 P9
  constraint midpoint L154 P10
  constraint coincident P10 L156.end
  constraint perpendicular L154 L157
  constraint coincident L157.end A139.centre
  constraint tangent A28 A139
  constraint concentric A139 A140
  constraint coincident P9 L158.end
  constraint perpendicular L155 L159
  constraint coincident L159.end A141.centre
  constraint tangent A25 A141
  constraint concentric A141 A142
  constraint coincident A143.centre L160.end
  constraint vertical L160
  constraint perpendicular L122 L161
  constraint coincident L161.end A144.centre
  measures "d1" diameter of A26
  measures "d2" angle of L1 L2
  measures "d3" angle of L1 L3
  measures "d4" distance of L5.end L6.end
  measures "d5" distance of L4.start L6.end
  measures "d6" diameter of A7
  measures "d7" distance of L5.end L8.end
  measures "d8" angle of L6 L8
  measures "d9" distance of L4.end L9.end
  measures "d10" angle of L4 L9
  measures "d11" diameter of A0
  measures "d12" distance of L13.start L13.end
  measures "d13" distance of L13.start L14.end
  measures "d14" diameter of A9
  measures "d15" diameter of A11
  measures "d16" distance of L14.end L17.end
  measures "d17" angle of L15 L17
  measures "d18" distance of L15.end L18.end
  measures "d19" angle of L15 L18
  measures "d21" distance of L22.start L22.end
  measures "d22" distance of L22.start L23.end
  measures "d23" diameter of A23
  measures "d24" diameter of A21
  measures "d25" distance of L24.end L26.end
  measures "d26" angle of L24 L26
  measures "d27" distance of L23.end L27.end
  measures "d28" angle of L24 L27
  measures "d29" distance of L31.end L32.end
  measures "d30" distance of L7 L32
  measures "d31" distance of L34.start L34.end
  measures "d32" distance of L34.start L36.end
  measures "d34" distance of L32 L35
  measures "d35" distance of L39.start L39.end
  measures "d36" distance of L39.start L41.end
  measures "d37" distance of L35 L42
  measures "d38" distance of L34.start L44.end
  measures "d39" distance of L34.end L45.end
  measures "d40" distance of L36.end L46.end
  measures "d41" distance of L35.end L47.end
  measures "d42" angle of L34 L44
  measures "d43" angle of L34 L45
  measures "d44" angle of L36 L46
  measures "d45" angle of L36 L47
  measures "d46" distance of L39.start L52.end
  measures "d47" distance of L39.end L53.end
  measures "d48" distance of L41.end L54.end
  measures "d49" distance of L40.end L55.end
  measures "d50" angle of L39 L52
  measures "d51" angle of L39 L53
  measures "d52" angle of L41 L54
  measures "d53" angle of L41 L55
  measures "d54" distance of L60.end L61.end
  measures "d55" distance of L13 L61
  measures "d56" distance of L63.end L64.end
  measures "d57" distance of L64.end L65.end
  measures "d58" distance of L61 L65
  measures "d59" distance of L68.end L69.end
  measures "d60" distance of L68.start L68.end
  measures "d61" distance of L65 L68
  measures "d62" distance of L65.end L73.end
  measures "d63" distance of L63.start L74.end
  measures "d64" distance of L63.end L76.end
  measures "d65" distance of L64.end L75.end
  measures "d66" angle of L63 L76
  measures "d67" angle of L65 L75
  measures "d68" angle of L65 L73
  measures "d69" angle of L63 L74
  measures "d70" distance of L70.end L81.end
  measures "d71" distance of L68.start L82.end
  measures "d72" distance of L69.end L83.end
  measures "d73" distance of L68.end L84.end
  measures "d74" angle of L68 L82
  measures "d75" angle of L70 L81
  measures "d76" angle of L70 L83
  measures "d77" angle of L68 L84
  measures "d78" distance of L89.end L90.end
  measures "d79" distance of L22 L90
  measures "d81" distance of L92.end L93.end
  measures "d82" distance of L92.start L92.end
  measures "d83" distance of L90 L94
  measures "d84" distance of L97.end L98.end
  measures "d85" distance of L98.end L99.end
  measures "d86" distance of L94 L97
  measures "d87" distance of L99.end L102.end
  measures "d88" distance of L97.start L103.end
  measures "d89" distance of L98.end L104.end
  measures "d90" distance of L97.end L105.end
  measures "d91" angle of L99 L102
  measures "d92" angle of L99 L104
  measures "d93" angle of L97 L105
  measures "d94" angle of L97 L103
  measures "d95" distance of L94.end L110.end
  measures "d96" distance of L92.start L111.end
  measures "d97" distance of L93.end L112.end
  measures "d98" distance of L92.end L113.end
  measures "d99" angle of L94 L110
  measures "d100" angle of L92 L111
  measures "d101" angle of L94 L112
  measures "d102" angle of L92 L113
  measures "d103" distance of L118.start L120.end
  measures "d104" distance of L0.start L121
  measures "d105" distance of L121 L125
  measures "d106" distance of L122.start L124.end
  measures "d107" distance of L125 L126
  measures "d108" distance of L122 L127.start
  measures "d109" angle of L122 L127
  measures "d110" distance of L124 L128.start
  measures "d111" angle of L124 L128
  measures "d112" distance of L120.end L129.end
  measures "d113" distance of L124.end L130.end
  measures "d114" angle of L120 L129
  measures "d115" angle of L124 L130
  measures "d116" diameter of A103
  measures "d117" distance of L118.start L131.end
  measures "d118" distance of L122.start L132.end
  measures "d119" angle of L118 L131
  measures "d120" angle of L122 L132
  measures "d121" diameter of A106
  measures "d122" diameter of A107
  measures "d123" diameter of A108
  measures "d124" diameter of A109
  measures "d125" diameter of A110
  measures "d131" diameter of A123
  measures "d132" diameter of A124
  measures "d133" diameter of A125
  measures "d134" diameter of A126
  measures "d135" diameter of A127
  measures "d136" diameter of A128
  measures "d137" diameter of A129
  measures "d138" diameter of A130
  measures "d139" diameter of A131
  measures "d140" diameter of A132
  measures "d141" diameter of A133
  measures "d142" diameter of A134
  measures "d143" diameter of A135
  measures "d144" diameter of A136
  measures "d145" diameter of A137
  measures "d146" diameter of A138
  measures "d147" diameter of A139
  measures "d148" diameter of A140
  measures "d149" diameter of A141
  measures "d150" diameter of A142
  measures "d189" diameter of A143
  measures "d190" distance of L126.end A143.centre
  measures "d191" distance of L126.start L161.end
  measures "d192" diameter of A144
  measures "d193" diameter of A145
  measures "d194" distance of L124 A145.centre
  measures "d195" distance of L91 A145.centre
  measures "d196" diameter of A146
  measures "d197" distance of L140 A146.centre
  measures "d198" distance of L62 A146.centre
extrude "Extrude1" add sketch "Sketch1" along normal blind 4.8
sketch "Sketch2" plane through (32, 0, 0) normal (1, 0, 0) x (0, 1, 0)
  line L0 (-16.1787, 0) -> (16.1787, 0)
  line L1 (16.1787, 0) -> (16.1787, 4.8)
  line L2 (16.1787, 4.8) -> (-16.1787, 4.8)
  line L3 (-16.1787, 4.8) -> (-16.1787, 0)
  line L4 (-16.1787, 4.8) -> (16.1787, 0) construction
  circle A0 centre (0, 2.4) radius 1.5
  point P0 (0, 2.4)
  dimension "d128" = 3
  constraint coincident L2.end L3.start
  constraint coincident L0.end L1.start
  constraint midpoint L4 P0
  constraint coincident P0 A0.centre
  measures "d128" diameter of A0
extrude "Extrude2" cut sketch "Sketch2" against normal blind 8 contours A0
thread "Thread1" "ISO Metric profile 3.0 M3x0.5 6H" major diameter 3.086 minor diameter 2.529 pitch 0.5 angle 60 modelled right hand crest width 0.1368 on face at (29.3333, 1.4925, 2.2506) crest through (31.875, 1.2645, 2.4)